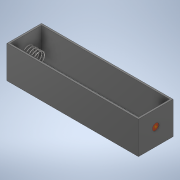
# Autodesk Inventor part: portapilas
Saved by Autodesk Inventor 2020 (Build 240168000, 168)
## iProperties
Created: 2022-02-15
Part Number: portapilas
Material: Genérico
Document SubType Name: Modeling
Designer: DANIEL
Density: 1 g/cm^3
Appearance: Suave - Negro
Author: DANIEL
Autodesk Inventor part; units mm, degrees
sketch "Boceto1" plane through (0, 0, 0) normal (0, 1, 0) x (-1, 0, 0)
  line L0 (38.5, 39.5) -> (-38.5, 39.5)
  line L1 (-38.5, 39.5) -> (-38.5, 19.75)
  line L2 (38.5, 19.75) -> (38.5, 39.5)
  line L3 (-38.5, 19.75) -> (-38.5, 0)
  line L4 (38.5, 0) -> (38.5, 19.75)
  line L5 (-38.5, 0) -> (-38.5, -19.75)
  line L6 (38.5, -19.75) -> (38.5, 0)
  line L7 (-38.5, -19.75) -> (-38.5, -39.5)
  line L8 (-38.5, -39.5) -> (38.5, -39.5)
  line L9 (38.5, -39.5) -> (38.5, -19.75)
  line L10 (38.5, 39.5) -> (-38.5, 39.5)
  line L11 (-38.5, 39.5) -> (-38.5, 38.5)
  line L12 (-37.5, 38.5) -> (37.5, 38.5)
  line L13 (38.5, 38.5) -> (38.5, 39.5)
  line L14 (37.5, 20.25) -> (-37.5, 20.25)
  line L15 (-38.5, 20.25) -> (-38.5, 19.25)
  line L16 (-37.5, 19.25) -> (37.5, 19.25)
  line L17 (38.5, 19.25) -> (38.5, 20.25)
  line L18 (37.5, 0.5) -> (-37.5, 0.5)
  line L19 (-38.5, 0.5) -> (-38.5, -0.5)
  line L20 (-37.5, -0.5) -> (37.5, -0.5)
  line L21 (38.5, -0.5) -> (38.5, 0.5)
  line L22 (37.5, -19.25) -> (-37.5, -19.25)
  line L23 (-38.5, -19.25) -> (-38.5, -20.25)
  line L24 (-37.5, -20.25) -> (37.5, -20.25)
  line L25 (38.5, -20.25) -> (38.5, -19.25)
  line L26 (38.5, -39.5) -> (-38.5, -39.5)
  line L27 (-38.5, -39.5) -> (-38.5, -38.5)
  line L28 (-37.5, -38.5) -> (37.5, -38.5)
  line L29 (38.5, -38.5) -> (38.5, -39.5)
  line L30 (38.5, 39.5) -> (37.5, 39.5)
  line L31 (37.5, -39.5) -> (38.5, -39.5)
  line L32 (38.5, -39.5) -> (38.5, 39.5)
  line L33 (-38.5, 39.5) -> (-37.5, 39.5)
  line L34 (-37.5, -39.5) -> (-38.5, -39.5)
  line L35 (-38.5, -39.5) -> (-38.5, 39.5)
  line L36 (37.5, 38.5) -> (37.5, 20.25)
  line L37 (37.5, 19.25) -> (37.5, 0.5)
  line L38 (37.5, -0.5) -> (37.5, -19.25)
  line L39 (37.5, -20.25) -> (37.5, -38.5)
  line L40 (-37.5, -20.25) -> (-37.5, -38.5)
  line L41 (-37.5, -0.5) -> (-37.5, -19.25)
  line L42 (-37.5, 38.5) -> (-37.5, 20.25)
  line L43 (-37.5, 19.25) -> (-37.5, 0.5)
  point P0 (0, 0)
  dimension "D" = 77
  dimension "P" = 19.75
  dimension "d2" = 19.75
  dimension "d3" = 19.75
  dimension "d4" = 19.75
  dimension "d6" = 38.5
  dimension "d18" = 1
  dimension "d19" = 1
  constraints: 88 end point, 24 parallel, 14 perpendicular, 13 point on line, 8 horizontal
  measures "D" distance of L2.start L1.end
  measures "P" distance of L1.end L0.end
  measures "d2" distance of L3.end L3.start
  measures "d3" distance of L5.end L5.start
  measures "d4" distance of L7.end L7.start
  measures "d6" distance from line of L1 point (0, 0)
  measures "d18" distance between parallel lines of L0 L12
  measures "d19" distance between parallel lines of L8 L28
extrude "Extrusión1" add sketch "Boceto1" along normal blind 18
sketch "Boceto2" plane through (0, 0, 0) normal (0, -1, 0) x (1, 0, 0)
  line L0 (38.5, -39.5) -> (-38.5, -39.5) projected
  line L1 (38.5, 39.5) -> (38.5, -39.5) projected
  line L2 (-38.5, -39.5) -> (-38.5, 39.5) projected
  line L3 (-38.5, 39.5) -> (38.5, 39.5) projected
  line L4 (38.5, -39.5) -> (-38.5, -39.5)
  line L5 (-38.5, -39.5) -> (-38.5, 39.5)
  line L6 (-38.5, 39.5) -> (38.5, 39.5)
  line L7 (38.5, 39.5) -> (38.5, -39.5)
  point P0 (0, 0)
  constraints: 8 end point, 2 parallel, 1 horizontal, 1 perpendicular
extrude "Extrusión2" add sketch "Boceto2" along normal blind 1
ref_plane "Plano de trabajo2" through (0, 9, 0) normal (0, 1, 0) x (1, 0, 0)
sketch "Boceto4" plane through (0, 9, 0) normal (0, 1, 0) x (1, 0, 0)
  line L0 (37.5, -38.5) -> (-37.5, -38.5) projected
  line L1 (-37.5, -38.5) -> (-37.5, -20.25) projected
  line L2 (-37.5, -20.25) -> (37.5, -20.25) projected
  line L3 (-37.5, -38.5) -> (-37.5, -20.25) projected
  line L4 (-37.5, -29.375) -> (-24.0433, -29.375)
  circle A0 centre (-37.5, -33.125) radius 0.25
  point P0 (0, 0)
  dimension "d28" = 0.5
  dimension "d29" = 4
  constraints: 2 end point, 1 centre point, 1 horizontal, 1 midpoint, 1 point on line
  measures "d28" diameter of A0
coil "Bobina1" sketch "Boceto4" operation add axis through (-37.5, 9, 29.375) along (1, 0, 0) pitch 1.6 turns 5 hand right
ref_plane "Plano de trabajo3" through (0, 9, 0) normal (0, 1, 0) x (1, 0, 0)
ref_plane "Plano de trabajo4" through (0, 9, 0) normal (0, 1, 0) x (1, 0, 0)
ref_plane "Plano de trabajo5" through (0, 9, 0) normal (0, 1, 0) x (1, 0, 0)
sketch "Boceto5" plane through (0.0276, 9, 39.2787) normal (0, 1, 0) x (-1, 0, 0)
  line L0 (37.5, -38.5) -> (-37.5, -38.5)
  line L1 (-37.5, -38.5) -> (-37.5, -20.25)
  line L2 (-37.5, -20.25) -> (37.5, -20.25)
  line L3 (-37.5, -38.5) -> (-37.5, -20.25)
  line L4 (-37.5, -29.375) -> (-24.0433, -29.375)
  circle A0 centre (-37.5, -33.125) radius 0.25
  point P0 (0, 0)
  dimension "d50" = 0.5
  dimension "d49" = 4
  constraints: 10 end point, 1 centre point, 1 horizontal, 1 midpoint, 1 point on line
  measures "d50" diameter of A0
coil "Bobina2" sketch "Boceto5" operation add axis through (37.5276, 9, 9.9037) along (-1, 0, 0) pitch 1.6 turns 5 hand right
sketch "Boceto6" plane through (-0.0956, 9, -39.5538) normal (0, 1, 0) x (1, 0, 0)
  line L0 (37.5, -38.5) -> (-37.5, -38.5)
  line L1 (-37.5, -38.5) -> (-37.5, -20.25)
  line L2 (-37.5, -20.25) -> (37.5, -20.25)
  line L3 (-37.5, -38.5) -> (-37.5, -20.25)
  line L4 (-37.5, -29.375) -> (-24.0433, -29.375)
  circle A0 centre (-37.5, -33.125) radius 0.25
  point P0 (0, 0)
  dimension "d60" = 0.5
  dimension "d59" = 4
  constraints: 10 end point, 1 centre point, 1 horizontal, 1 midpoint, 1 point on line
  measures "d60" diameter of A0
coil "Bobina3" sketch "Boceto6" operation add axis through (-37.5956, 9, -10.1788) along (1, 0, 0) pitch 1.6 turns 5 hand right
sketch "Boceto7" plane through (0.0336, 9, -0.0217) normal (0, 1, 0) x (-1, 0, 0)
  line L0 (37.5, -38.5) -> (-37.5, -38.5)
  line L1 (-37.5, -38.5) -> (-37.5, -20.25)
  line L2 (-37.5, -20.25) -> (37.5, -20.25)
  line L3 (-37.5, -38.5) -> (-37.5, -20.25)
  line L4 (-37.5, -29.375) -> (-24.0433, -29.375)
  circle A0 centre (-37.5, -33.125) radius 0.25
  point P0 (0, 0)
  dimension "d70" = 0.5
  dimension "d69" = 4
  constraints: 10 end point, 1 centre point, 1 horizontal, 1 midpoint, 1 point on line
  measures "d70" diameter of A0
coil "Bobina4" sketch "Boceto7" operation add axis through (37.5336, 9, -29.3967) along (-1, 0, 0) pitch 1.6 turns 5 hand right
sketch "Boceto8" plane through (38.5, 18, 39.5) normal (1, 0, 0) x (0, 0, -1)
  circle A0 centre (3, -2) radius 0.75
  circle A1 centre (6, -2) radius 0.75
  line L0 (0, 0) -> (79, 0) projected
  line L1 (0, 0) -> (0, -19) projected
  point P0 (39.5, -18)
  dimension "d71" = 1.5
  dimension "d72" = 1.5
  dimension "d73" = 3
  dimension "d74" = 2
  dimension "d88" = 3
  constraints: 2 centre point, 1 horizontal alignment
  measures "d71" diameter of A0
  measures "d72" diameter of A1
  measures "d73" distance of A1.centre A0.centre
  measures "d74" distance from line of L0 A0.centre
  measures "d88" distance from line of L1 A0.centre
extrude "Extrusión3" [suppressed]
sketch "Boceto9" plane through (38.5, 18, 39.5) normal (1, 0, 0) x (0, 0, -1)
  line L0 (79, -19) -> (0, -19) projected
  line L1 (0, -19) -> (0, 0) projected
  line L2 (0, 0) -> (79, 0) projected
  line L3 (79, 0) -> (79, -19) projected
  line L4 (1, -18) -> (1, 0) projected
  line L5 (19.25, -18) -> (1, -18) projected
  line L6 (19.25, -18) -> (19.25, 0) projected
  line L7 (20.25, -18) -> (20.25, 0) projected
  line L8 (39, -18) -> (20.25, -18) projected
  line L9 (40, -18) -> (40, 0) projected
  line L10 (39, -18) -> (39, 0) projected
  line L11 (58.75, -18) -> (40, -18) projected
  line L12 (58.75, -18) -> (58.75, 0) projected
  line L13 (59.75, -18) -> (59.75, 0) projected
  line L14 (78, -18) -> (59.75, -18) projected
  line L15 (78, -18) -> (78, 0) projected
  circle A0 centre (10.125, -9) radius 2
  circle A1 centre (29.375, -9) radius 2
  circle A2 centre (49.125, -9) radius 2
  circle A3 centre (68.875, -9) radius 2
  point P0 (39.5, -18)
  dimension "d77" = 4
  dimension "d78" = 4
  dimension "d79" = 4
  dimension "d80" = 4
  dimension "d81" = 9
  dimension "d82" = 9.125
  dimension "d83" = 9.125
  dimension "d84" = 9.125
  dimension "d85" = 9.125
  constraints: 4 centre point, 3 horizontal alignment, 1 other
  measures "d77" diameter of A0
  measures "d78" diameter of A1
  measures "d79" diameter of A2
  measures "d80" diameter of A3
  measures "d82" distance from line of L4 A0.centre
  measures "d83" distance from line of L7 A1.centre
  measures "d84" distance from line of A2.centre L9
  measures "d85" distance from line of L13 A3.centre
extrude "Extrusión4" cut sketch "Boceto9" against normal blind 0.25 contours A0 | A1 | A2 | A3
sketch "Boceto10" plane through (38.5, 18, 39.5) normal (1, 0, 0) x (0, 0, -1)
  circle A0 centre (3, -2) radius 0.75 projected
sketch "Boceto11" plane through (38.5, 18, 39.5) normal (1, 0, 0) x (0, 0, -1)
  circle A0 centre (6, -2) radius 0.75 projected
sketch "Boceto12" plane through (38.5, 18, 39.5) normal (1, 0, 0) x (0, 0, -1)
  circle A0 centre (10.125, -9) radius 2 projected
sketch "Boceto13" plane through (38.5, 18, 39.5) normal (1, 0, 0) x (0, 0, -1)
  circle A0 centre (49.125, -9) radius 2 projected
sketch "Boceto14" plane through (38.5, 18, 39.5) normal (1, 0, 0) x (0, 0, -1)
  circle A0 centre (29.375, -9) radius 2 projected
sketch "Boceto15" plane through (38.5, 18, 39.5) normal (1, 0, 0) x (0, 0, -1)
  circle A0 centre (68.875, -9) radius 2 projected
sketch "Boceto16" plane through (-38.5, 18, -39.5) normal (-1, 0, 0) x (0, 0, 1)
  line L0 (0, -19) -> (0, 0) projected
  line L1 (1, -18) -> (1, 0) projected
  line L2 (19.25, -18) -> (19.25, 0) projected
  line L3 (20.25, -18) -> (20.25, 0) projected
  line L4 (19.25, -18) -> (1, -18) projected
  line L5 (39, -18) -> (20.25, -18) projected
  line L6 (40, -18) -> (40, 0) projected
  line L7 (39, -18) -> (39, 0) projected
  line L8 (79, -19) -> (0, -19) projected
  line L9 (58.75, -18) -> (40, -18) projected
  line L10 (59.75, -18) -> (59.75, 0) projected
  line L11 (58.75, -18) -> (58.75, 0) projected
  line L12 (78, -18) -> (59.75, -18) projected
  line L13 (79, -19) -> (79, 0) projected
  line L14 (78, -18) -> (78, 0) projected
  line L15 (0, 0) -> (79, 0) projected
  circle A0 centre (10.125, -9) radius 2
  circle A1 centre (29.875, -9) radius 2 projected
  circle A2 centre (49.625, -9) radius 2 projected
  circle A3 centre (68.875, -9) radius 2 projected
  circle A4 centre (29.875, -9) radius 2
  circle A5 centre (49.625, -9) radius 2
  circle A6 centre (68.875, -9) radius 2
  point P0 (39.5, -18)
  dimension "d89" = 4
  constraints: 4 centre point, 3 coincident, 3 concentric, 1 other
  measures "d89" diameter of A0
extrude "Extrusión5" cut sketch "Boceto16" against normal blind 0.25 contours A0 | A1 | A2 | A3
sketch "Boceto17" plane through (-38.5, 18, -39.5) normal (-1, 0, 0) x (0, 0, 1)
  circle A0 centre (68.875, -9) radius 2 projected
sketch "Boceto18" plane through (-38.5, 18, -39.5) normal (-1, 0, 0) x (0, 0, 1)
  circle A0 centre (49.625, -9) radius 2 projected
sketch "Boceto19" plane through (-38.5, 18, -39.5) normal (-1, 0, 0) x (0, 0, 1)
  circle A0 centre (29.875, -9) radius 2 projected
sketch "Boceto20" plane through (-38.5, 18, -39.5) normal (-1, 0, 0) x (0, 0, 1)
  circle A0 centre (10.125, -9) radius 2 projected
sketch "Boceto21" plane through (37.5, 18, 19.25) normal (0, 0, -1) x (-1, 0, 0)
  line L0 (79.057, 4.0056) -> (-4.5478, 4.0056)
  line L1 (-4.5478, 4.0056) -> (-4.5478, -24.6262)
  line L2 (-4.5478, -24.6262) -> (79.057, -24.6262)
  line L3 (79.057, -24.6262) -> (79.057, 4.0056)
  point P0 (37.5, -18)
  constraints: 8 end point, 2 parallel, 1 horizontal, 1 perpendicular
extrude "Extrusión6" cut sketch "Boceto21" along normal blind 67
equation "\"d2\" = P"
equation "\"d3\" = P"
equation "\"d4\" = P"
equation "\"d6\" = 0.5 * D"
equation "\"d10\" = Q"
equation "\"Q\" = 0.5"
